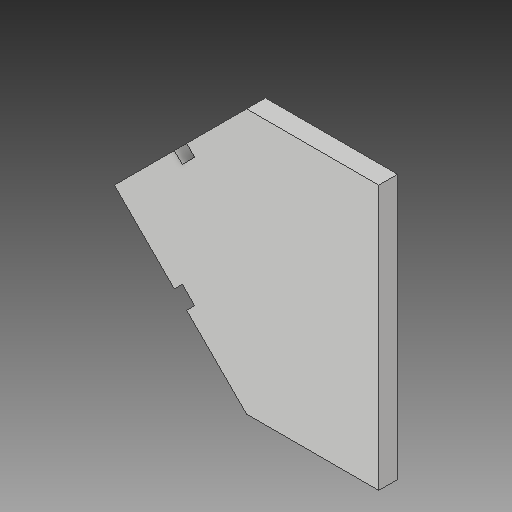
# Autodesk Inventor part: frame1
Saved by Autodesk Inventor 2019 (Build 230136000, 136)
## iProperties
Created: 2020-03-15
Part Number: frame1
Material: Generic
Document SubType Name: Modeling
Designer: Pulag
Mass: 18.2359 g
Surface Area: 85.4934 cm^2
Volume: 18.2359 cm^3
Density: 1 g/cm^3
Appearance: Default
Author: Pulag
Autodesk Inventor part; units mm, degrees
ref_plane "YZ Plane" through (0, 0, 0) normal (1, 0, 0) x (0, 1, 0)
ref_plane "XZ Plane" through (0, 0, 0) normal (0, 1, 0) x (-1, 0, 0)
ref_plane "XY Plane" through (0, 0, 0) normal (0, 0, 1) x (1, 0, 0)
sketch "Sketch1" plane through (0, 0, 0) normal (0, 0, 1) x (1, 0, 0)
  line L0 (0, 35) -> (35, 35)
  line L1 (35, 35) -> (35, -35)
  line L2 (0, -35) -> (-35, 0)
  line L3 (0, 35) -> (-35, 0)
  line L4 (35, -35) -> (0, -35)
  point P0 (0, 0)
  dimension "d1" = 70
  constraints: 10 end point, 2 horizontal, 1 perpendicular
  measures "d1" distance of L0.end L1.end
extrude "Extrusion1" add sketch "Sketch1" along normal blind 5
sketch "Sketch2" plane through (0, 0, 5) normal (0, 0, 1) x (1, 0, 0)
  line L0 (0, 35) -> (-35, 0) projected
  line L1 (-35, 0) -> (0, -35) projected
  line L2 (-13.7396, 17.0178) -> (-15.8609, 19.1391)
  line L3 (-17.0178, 13.7396) -> (-19.1391, 15.8609)
  line L4 (-13.7396, 17.0178) -> (-17.0178, 13.7396)
  line L5 (0, 0) -> (-35, 0)
  line L6 (-13.7396, -17.0178) -> (-15.8609, -19.1391)
  line L7 (-17.0178, -13.7396) -> (-19.1391, -15.8609)
  line L8 (-13.7396, -17.0178) -> (-17.0178, -13.7396)
  line L9 (-15.8609, 19.1391) -> (-19.1391, 15.8609)
  line L10 (-19.1391, -15.8609) -> (-15.8609, -19.1391)
  dimension "d6" = 4.636
  constraints: 18 end point, 4 symmetric about line, 2 collinear, 2 point on line, 1 horizontal, 1 perpendicular
  measures "d6" distance of L3.start L2.start
extrude "Extrusion2" cut sketch "Sketch2" against normal blind 5
body "Solid1"
